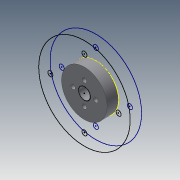
# Autodesk Inventor part: pulleyFlange
Saved by Autodesk Inventor 2015 (Build 190159000, 159)
## iProperties
Created: 2014-09-01
Part Number: pulleyFlange
Material: Generic
Document SubType Name: Modeling
Designer: shohei
Density: 1 g/cm^3
Appearance: Default
Author: shohei
Autodesk Inventor part; units mm, degrees
ref_plane "YZ Plane" through (0, 0, 0) normal (1, 0, 0) x (0, 1, 0)
ref_plane "XZ Plane" through (0, 0, 0) normal (0, 1, 0) x (-1, 0, 0)
ref_plane "XY Plane" through (0, 0, 0) normal (0, 0, 1) x (1, 0, 0)
sketch "Block1" plane through (0, 0, 0) normal (0, 0, 1) x (1, 0, 0)
  circle A0 centre (0, 0) radius 40.22
  circle A1 centre (30, -0.0076) radius 2.22
  circle A2 centre (0.0076, 30) radius 2.22
  circle A3 centre (0, 0) radius 5.22
  circle A4 centre (-30, 0.0076) radius 2.22
  circle A5 centre (-0.0076, -30) radius 2.22
  point P0 (0, 0)
sketch "Block2" plane through (0, 0, 0) normal (0, 0, 1) x (1, 0, 0)
  circle A0 centre (0, 0) radius 20.22
  circle A1 centre (10, -0.0076) radius 2.22
  circle A2 centre (0.0076, 10) radius 2.22
  circle A3 centre (0, 0) radius 5.22
  circle A4 centre (-0.0076, -10) radius 2.22
  circle A5 centre (-10, 0.0076) radius 2.22
  point P0 (0, 0)
sketch "Sketch1" plane through (0, 0, 0) normal (0, 1, 0) x (-1, 0, 0)
  circle A0 centre (0, 0) radius 20
  circle A1 centre (10, -0.0076) radius 2
  circle A2 centre (0, 0) radius 5
  arc A3 (-36.0813, 0.572) -> (-36.0815, -0.5576) centre (0, 0) ccw
  arc A4 (-0.0152, -40) -> (-0.0008, -40) centre (0, 0) ccw
  arc A5 (-0.5728, -36.0815) -> (0.5584, -36.0818) centre (0, 0) ccw
  circle A6 centre (0.0076, 10) radius 2
  circle A7 centre (-10, 0.0076) radius 2
  circle A8 centre (-0.0076, -10) radius 2
  point P0 (12, -0.0008)
  point P1 (8.0813, -0.572)
  point P2 (-36.0815, 0.5728)
  point P3 (-0.5576, 36.0815)
  point P4 (0.572, 36.0813)
  point P5 (0.0008, 12)
  point P6 (0.572, 8.0813)
  point P7 (0.5576, -36.0815)
  point P8 (-12, 0.0008)
  point P9 (-8.0813, 0.572)
  point P10 (36.0815, 0.5576)
  point P11 (-0.0008, -12)
  point P12 (-0.572, -8.0813)
  point P13 (-0.5576, 36.0815)
  dimension "d0" = 40
  dimension "d2" = 4
  dimension "d7" = 10
  dimension "d12" = 10
  dimension "d15" = 360
  constraints: 14 point on circle, 9 centre point, 3 coincident, 21 other
  measures "d0" diameter of A0
  measures "d2" diameter of A1
  measures "d7" diameter of A2
  measures "d12" distance of A1.centre A2.centre
extrude "Extrusion2" add sketch "Sketch1" along normal blind 10
sketch "Sketch4" plane through (0, 10, 0) normal (0, 1, 0) x (1, 0, 0)
  circle A0 centre (0, 0) radius 5 projected
  circle A1 centre (0.0076, 10) radius 2 projected
  circle A2 centre (10, -0.0076) radius 2 projected
  circle A3 centre (-0.0076, -10) radius 2 projected
  circle A4 centre (-10, 0.0076) radius 2 projected
  circle A5 centre (0, 0) radius 20 projected
  circle A6 centre (0, 0) radius 20.22
  circle A7 centre (10, -0.0076) radius 2.22
  circle A8 centre (0.0076, 10) radius 2.22
  circle A9 centre (0, 0) radius 5.22
  circle A10 centre (-0.0076, -10) radius 2.22
  circle A11 centre (-10, 0.0076) radius 2.22
  constraints: 6 other
sketch "DXF" plane through (0, 0, 0) normal (0, 1, 0) x (-1, 0, 0)
  circle A0 centre (0, 0) radius 20.22
  circle A1 centre (10, -0.0076) radius 2.22
  circle A2 centre (0.0076, 10) radius 2.22
  circle A3 centre (0, 0) radius 5.22
  circle A4 centre (-0.0076, -10) radius 2.22
  circle A5 centre (-10, 0.0076) radius 2.22
body "Solid2"
